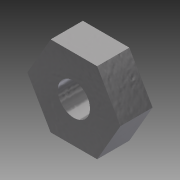
# Autodesk Inventor part: Nut
Saved by Autodesk Inventor 2015 (Build 190159000, 159)
## iProperties
Created: 2016-01-20
Part Number: Nut
Material: Generic
Document SubType Name: Modeling
Designer: Kyle
Density: 1 g/cm^3
Appearance: Galvanized
Author: Kyle
Autodesk Inventor part; units mm, degrees
ref_plane "YZ Plane" through (0, 0, 0) normal (1, 0, 0) x (0, 1, 0)
ref_plane "XZ Plane" through (0, 0, 0) normal (0, 1, 0) x (-1, 0, 0)
ref_plane "XY Plane" through (0, 0, 0) normal (0, 0, 1) x (1, 0, 0)
sketch "Sketch1" plane through (0, 0, 0) normal (0, 0, 1) x (1, 0, 0)
  line L0 (-1.8331, 3.175) -> (1.8331, 3.175)
  line L1 (1.8331, 3.175) -> (3.6662, 0)
  line L2 (3.6662, 0) -> (1.8331, -3.175)
  line L3 (1.8331, -3.175) -> (-1.8331, -3.175)
  line L4 (-1.8331, -3.175) -> (-3.6662, 0)
  line L5 (-3.6662, 0) -> (-1.8331, 3.175)
  circle A0 centre (0, 0) radius 1.27
  dimension "d0" = 6.35
  dimension "d1" = 2.54
  constraints: 12 end point, 2 coincident, 1 centre point, 1 horizontal, 13 other
  measures "d0" distance between parallel lines of L1 L4
  measures "d1" diameter of A0
extrude "Extrusion1" add sketch "Sketch1" along normal blind 2.54
body "Solid1"
